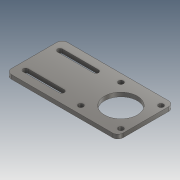
# Autodesk Inventor part: nema_support_1
Saved by Autodesk Inventor 2017 (Build 210142000, 142)
## iProperties
Created: 2018-05-19
Part Number: nema_support_1
Material: Steel, Carbon
Document SubType Name: Sheet Metal
Designer: Luiz Gustavo
Density: 7.85 g/cm^3
Sheet Metal Rule: Default_mm
Appearance: Semi-Polished
Author: Luiz Gustavo
Autodesk Inventor part; units mm, degrees
ref_plane "YZ Plane" through (0, 0, 0) normal (1, 0, 0) x (0, 1, 0)
ref_plane "XZ Plane" through (0, 0, 0) normal (0, 1, 0) x (-1, 0, 0)
ref_plane "XY Plane" through (0, 0, 0) normal (0, 0, 1) x (1, 0, 0)
sketch "Sketch1" plane through (0, 0, 0) normal (0, 0, 1) x (1, 0, 0)
  circle A0 centre (0, 0) radius 33 construction
  circle A1 centre (0, 0) radius 19.1
  line L0 (-101, -32.5) -> (29, -32.5)
  line L1 (29, -32.5) -> (29, 32.5)
  line L2 (29, 32.5) -> (-101, 32.5)
  line L3 (-101, 32.5) -> (-101, -32.5)
  line L4 (-101, -32.5) -> (29, 32.5) construction
  line L5 (29, -32.5) -> (-101, 32.5) construction
  line L6 (-101, 0) -> (29, 0) construction
  arc A2 (-91, 23) -> (-91, 17) centre (-91, 20) ccw
  line L7 (-91, 20) -> (-49, 20) construction
  arc A3 (-52, 20) -> (-49, 17) centre (-49, 20) ccw construction
  line L8 (-91, 23) -> (-49, 23)
  line L9 (-91, 17) -> (-49, 17)
  arc A4 (-88, 20) -> (-91, 23) centre (-91, 20) ccw construction
  arc A5 (-91, 17) -> (-88, 20) centre (-91, 20) ccw construction
  arc A6 (-49, 23) -> (-52, 20) centre (-49, 20) ccw construction
  arc A7 (-49, 17) -> (-49, 23) centre (-49, 20) ccw
  arc A8 (-91, -17) -> (-91, -23) centre (-91, -20) ccw
  line L10 (-91, -23) -> (-49, -23)
  line L11 (-91, -17) -> (-49, -17)
  arc A9 (-49, -23) -> (-49, -17) centre (-49, -20) ccw
  line L12 (23.3345, -23.3345) -> (-23.3345, 23.3345) construction
  line L13 (-23.3345, -23.3345) -> (23.3345, 23.3345) construction
  circle A10 centre (23.3345, 23.3345) radius 3
  circle A11 centre (-23.3345, 23.3345) radius 3
  circle A12 centre (-23.3345, -23.3345) radius 3
  circle A13 centre (23.3345, -23.3345) radius 3
  point P0 (-36, 0)
  dimension "d0" = 66
  dimension "d1" = 38.2
  dimension "d2" = 130
  dimension "d3" = 65
  dimension "d4" = 101
  dimension "d5" = 6
  dimension "d6" = 10
  dimension "d7" = 52
  dimension "d8" = 40
  dimension "d9" = 45
  measures "d0" diameter of A0
  measures "d1" diameter of A1
  measures "d2" distance of L2.end L1.end
  measures "d3" distance of L1.end L0.end
  measures "d4" distance from line of point (0, 0) L3
  measures "d5" diameter of A2
  measures "d6" distance from line of L3 L7.start
  measures "d7" distance from line of L7.end L3
  measures "d8" distance of A8.centre L7.start
  measures "d9" angle of L6 L12
extrude "Plate1" add sketch "Sketch1" along normal blind 4.75
fillet "Corner Round1" radius 6 4 edges at (29, 32.5, 2.375) (29, -32.5, 2.375) (-101, -32.5, 2.375) (-101, 32.5, 2.375)
equation "\"BendRadius\" = Thickness"
equation "\"BendReliefWidth\" = Thickness"
equation "\"BendReliefDepth\" = 0.5 * Thickness"
equation "\"CornerReliefSize\" = 4 * Thickness"
equation "\"MinimumRemnant\" = 2 * Thickness"
equation "\"TransitionRadius\" = BendRadius"
equation "\"JacobiRadiusSize\" = BendRadius"
equation "\"GapSize\" = Thickness"
equation "\"d10\" = BendRadius"
equation "\"Thickness\" = 4.75"
body "Solid1"
